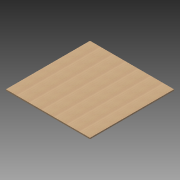
# Autodesk Inventor part: Boden
Saved by Autodesk Inventor 2013 SP1 (Build 170176100, 176)
## iProperties
Created: 2012-12-08
Part Number: Boden
Material: Esche
Document SubType Name: Modeling
Designer: Sebastian
Density: 1 g/cm^3
Author: Sebastian
Autodesk Inventor part; units mm, degrees
ref_plane "YZ Plane" through (0, 0, 0) normal (1, 0, 0) x (0, 1, 0)
ref_plane "XZ Plane" through (0, 0, 0) normal (0, 1, 0) x (-1, 0, 0)
ref_plane "XY Plane" through (0, 0, 0) normal (0, 0, 1) x (1, 0, 0)
sketch "Skizze1" plane through (0, 0, 0) normal (0, 0, 1) x (1, 0, 0)
  line L0 (-201, -201) -> (201, -201)
  line L1 (201, -201) -> (201, 201)
  line L2 (201, 201) -> (-201, 201)
  line L3 (-201, 201) -> (-201, -201)
  line L4 (-201, -201) -> (201, 201) construction
  line L5 (201, -201) -> (-201, 201) construction
  point P0 (0, 0)
  dimension "d0" = 402
  dimension "d1" = 402
  constraints: 12 end point, 2 midpoint, 2 parallel, 1 horizontal, 1 perpendicular
  measures "d0" distance of L2.end L1.end
  measures "d1" distance of L1.end L0.end
extrude "Extrusion1" add sketch "Skizze1" against normal blind 6
